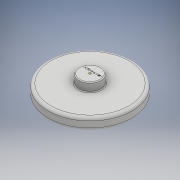
# Autodesk Inventor part: 前輪
Saved by Autodesk Inventor 2018 (Build 220112000, 112)
## iProperties
Created: 2017-09-09
Part Number: 前輪
Material: 一般
Document SubType Name: Modeling
Designer: Kenta
Density: 1 g/cm^3
Appearance: 既定
Author: Kenta
Autodesk Inventor part; units mm, degrees
ref_plane "YZ Plane" through (0, 0, 0) normal (1, 0, 0) x (0, 1, 0)
ref_plane "XZ Plane" through (0, 0, 0) normal (0, 1, 0) x (-1, 0, 0)
ref_plane "XY Plane" through (0, 0, 0) normal (0, 0, 1) x (1, 0, 0)
sketch "スケッチ1" plane through (0, 0, 0) normal (0, 0, 1) x (1, 0, 0)
  circle A0 centre (0, 0) radius 245
  dimension "d0" = 490
  constraints: 1 centre point, 1 coincident
  measures "d0" diameter of A0
extrude "押し出し1" add sketch "スケッチ1" along normal mid plane 70
fillet "フィレット1" radius 17.5 2 edges at (-245, 0, 35) (-245, 0, -35)
sketch "スケッチ8" plane through (0, 0, 35) normal (0, 0, 1) x (1, 0, 0)
  circle A0 centre (0, 0) radius 64
  dimension "d11" = 128
  constraints: 1 centre point, 1 coincident
  measures "d11" diameter of A0
extrude "押し出し2" add sketch "スケッチ8" along normal blind 50
sketch "スケッチ9" plane through (0, 0, -35) normal (0, 0, -1) x (-1, 0, 0)
  circle A0 centre (0, 0) radius 108
  dimension "d14" = 216
  constraints: 1 centre point, 1 coincident
  measures "d14" diameter of A0
extrude "押し出し3" add sketch "スケッチ9" along normal blind 48
fillet "フィレット2" radius 5 1 edges at (-64, 0, 85)
fillet "フィレット3" radius 5 1 edges at (-64, 0, 35)
fillet "フィレット4" radius 5 2 edges at (108, 0, -83) (108, 0, -35)
sketch "スケッチ10" plane through (0, 0, -83) normal (0, 0, -1) x (-1, 0, 0)
  point P0 (0, 0)
  point P1 (0, 0)
  constraints: 1 coincident
hole "穴2" at (0, 0, -83) direction (0, 0, 1) diameter 12 end through all
sketch "スケッチ12" plane through (0, 0, 85) normal (0, 0, 1) x (1, 0, 0)
  line L0 (-51.2549, 22.4229) -> (29.3453, 22.4229) construction
  line L1 (29.3453, 22.4229) -> (29.3453, -28.267) construction
  line L2 (29.3453, -28.267) -> (-51.2549, -28.267) construction
  line L3 (-51.2549, -28.267) -> (-51.2549, 22.4229) construction
  point P0 (0, 0)
  constraints: 2 other
sketch "スケッチ13" plane through (0, 0, -83) normal (0, 0, -1) x (-1, 0, 0)
  line L0 (-79.0903, 45.7594) -> (75.7007, 45.7594) construction
  line L1 (75.7007, 45.7594) -> (75.7007, -24.292) construction
  line L2 (75.7007, -24.292) -> (-79.0903, -24.292) construction
  line L3 (-79.0903, -24.292) -> (-79.0903, 45.7594) construction
  point P0 (0, 0)
  constraints: 2 other
sketch "スケッチ14" plane through (0, 0, -35) normal (0, 0, -1) x (-1, 0, 0)
  line L0 (-67.9, 178.6198) -> (94.9078, 178.6198) construction
  line L1 (94.9078, 178.6198) -> (94.9078, 134.9225) construction
  line L2 (94.9078, 134.9225) -> (-67.9, 134.9225) construction
  line L3 (-67.9, 134.9225) -> (-67.9, 178.6198) construction
  point P0 (0, 0)
  constraints: 2 other
